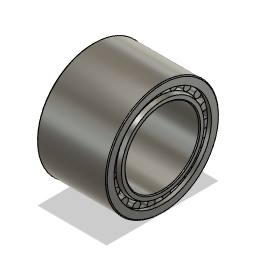
Bearing_GOST_7634-75_452000 (Autodesk Fusion 360 design; units mm, degrees)
Autodesk Fusion 360 part; units mm, degrees
note: some values were not read from the file. Chosen so that the rebuilt part matches the saved one: which bodies a step acts on.
sketch "Sketch1" plane through (0, 0, 0) normal (0, 0, 1) x (1, 0, 0)
  line L0 (-45.3984, 0) -> (45.3984, 0)
  line L1 (-80, 130) -> (80, 130)
  line L2 (80, 130) -> (80, 116.5)
  line L3 (80, 116.5) -> (-80, 116.5)
  line L4 (-80, 116.5) -> (-80, 130)
  line L5 (-80, 116.5) -> (-70.8611, 116.5)
  line L6 (-70.8611, 116.5) -> (-70.8611, 112)
  line L7 (-70.8611, 112) -> (-80, 112)
  line L8 (-80, 112) -> (-80, 116.5)
  line L9 (80, 116.5) -> (70.8611, 116.5)
  line L10 (70.8611, 116.5) -> (70.8611, 112)
  line L11 (70.8611, 112) -> (80, 112)
  line L12 (80, 112) -> (80, 116.5)
  line L13 (-80, 85) -> (80, 85)
  line L14 (-80, 85) -> (-80, 95.1737)
  line L15 (-80, 95.1737) -> (-70.8611, 98.5)
  line L16 (-70.8611, 98.5) -> (70.8611, 98.5)
  line L17 (80, 85) -> (80, 95.1737)
  line L18 (80, 95.1737) -> (70.8611, 98.5)
  line L19 (-70.8611, 98.5) -> (-70.8611, 112)
  line L20 (70.8611, 98.5) -> (70.8611, 112)
  line L21 (0, 98.5) -> (0, 85) construction
  line L22 (-70.8611, 107.5) -> (70.8611, 107.5)
  line L23 (-53.5833, 116.5) -> (-53.5833, 98.5)
  line L24 (0, 116.5) -> (0, 98.5)
  line L25 (-53.0833, 116.5) -> (-53.0833, 98.5)
  line L26 (-35.8056, 116.5) -> (-35.8056, 98.5)
  line L27 (-35.3056, 116.5) -> (-35.3056, 98.5)
  line L28 (-18.0278, 116.5) -> (-18.0278, 98.5)
  line L29 (-17.5278, 116.5) -> (-17.5278, 98.5)
  line L30 (-0.25, 116.5) -> (-0.25, 98.5)
  line L31 (0, 116.5) -> (0, 98.5)
  line L32 (17.5278, 116.5) -> (17.5278, 98.5)
  line L33 (18.0278, 116.5) -> (18.0278, 98.5)
  line L34 (35.3056, 116.5) -> (35.3056, 98.5)
  line L35 (35.8056, 116.5) -> (35.8056, 98.5)
  line L36 (53.0833, 116.5) -> (53.0833, 98.5)
  line L37 (53.5833, 116.5) -> (53.5833, 98.5)
  line L38 (0.25, 116.5) -> (0.25, 98.5)
  point P0 (0, 130)
  point P1 (0, 107.5)
  point P2 (0, 107.5)
  dimension "d1" = 170
  dimension "d2" = 20
  dimension "d3" = 20
  dimension "d4" = 260
  dimension "d5" = 160
  dimension "d7" = 18
  dimension "d8" = 9.1389
  dimension "d9" = 9
  dimension "d10" = 17.2778
  dimension "d23" = 0.5
  dimension "d24" = 17.2778
  dimension "d25" = 0.5
  dimension "d26" = 17.2778
  dimension "d27" = 0.5
  dimension "d28" = 17.2778
  dimension "d30" = 0.5
  dimension "d31" = 17.2778
  dimension "d32" = 0.5
  dimension "d33" = 17.2778
  dimension "d34" = 0.5
  dimension "d35" = 0.5
  dimension "d36" = 17.2778
  constraint horizontal L0
  constraint midpoint L0 origin
  constraint horizontal L1
  constraint vertical L2
  constraint horizontal L3
  constraint vertical L4
  constraint horizontal L5
  constraint vertical L6
  constraint horizontal L7
  constraint vertical L8
  constraint horizontal L9
  constraint vertical L10
  constraint horizontal L11
  constraint vertical L12
  constraint midpoint L1 P0
  constraint vertical origin P0
  constraint equal L7 L11
  constraint horizontal L13
  constraint vertical L1.end L13.end
  constraint vertical L1.start L13.start
  constraint perpendicular L13 L14
  constraint perpendicular L14 L16
  constraint perpendicular L13 L17
  constraint vertical L6.end L15.end
  constraint vertical L10.end L16.end
  constraint perpendicular L16 L19
  constraint perpendicular L11 L20
  constraint horizontal L6.end L10.end
  constraint midpoint L16 L21.start
  constraint midpoint L13 L21.end
  constraint equal L4 L21
  constraint coincident L22 P2
  constraint coincident L20 L22.end
  constraint coincident L19 L22.start
  constraint coincident L3 L23.start
  constraint coincident L16 L23.end
  constraint perpendicular L16 L23
  constraint midpoint L22 P2
  constraint midpoint L3 L24.start
  constraint midpoint L24 P2
  constraint coincident P2 P1
  constraint coincident L3 L25.start
  constraint coincident L16 L25.end
  constraint perpendicular L16 L25
  constraint coincident L3 L26.start
  constraint coincident L16 L26.end
  constraint perpendicular L16 L26
  constraint coincident L3 L27.start
  constraint coincident L16 L27.end
  constraint perpendicular L3 L27
  constraint coincident L3 L28.start
  constraint coincident L16 L28.end
  constraint perpendicular L16 L28
  constraint coincident L3 L29.start
  constraint coincident L16 L29.end
  constraint perpendicular L3 L29
  constraint coincident L3 L30.start
  constraint coincident L16 L30.end
  constraint perpendicular L16 L30
  constraint coincident L3 L24.start
  constraint coincident L16 L21.start
  constraint perpendicular L16 L31
  constraint coincident L24.start L31.start
  constraint coincident L3 L32.start
  constraint coincident L16 L32.end
  constraint perpendicular L16 L32
  constraint coincident L3 L33.start
  constraint coincident L16 L33.end
  constraint perpendicular L16 L33
  constraint coincident L3 L34.start
  constraint coincident L16 L34.end
  constraint perpendicular L16 L34
  constraint coincident L3 L35.start
  constraint coincident L16 L35.end
  constraint perpendicular L16 L35
  constraint coincident L3 L36.start
  constraint coincident L16 L36.end
  constraint perpendicular L16 L36
  constraint coincident L3 L37.start
  constraint coincident L16 L37.end
  constraint perpendicular L16 L37
  constraint coincident L3 L38.start
  constraint coincident L16 L38.end
  constraint perpendicular L16 L38
  measures "d2" angle of L16 L18
  measures "d3" angle of L15 L16
  measures "d5" distance of L1.start L1.end
  measures "d7" distance of L3 L16
  measures "d8" distance of L6.end L7.end
  measures "d10" distance of L19 L23
  measures "d23" distance of L23 L25
  measures "d24" distance of L25 L26
  measures "d25" distance of L26 L27
  measures "d26" distance of L27 L28
  measures "d27" distance of L28 L29
  measures "d28" distance of L29 L30
  measures "d30" distance of L32 L33
  measures "d31" distance of L33 L34
  measures "d32" distance of L34 L35
  measures "d33" distance of L35 L36
  measures "d34" distance of L36 L37
  measures "d35" distance of L30 L38
  measures "d36" distance of L32 L38
revolve "Revolve1" add sketch "Sketch1" angle 360 about axis through (-45.3984, 0, 0) along (1, 0, 0) contours L1 L2 L3 L4 L5 L9 | L3 L5 L6 L7 L8 | L3 L9 L10 L11 L12 | L13 L14 L15 L16 L17 L18 makes body 1 at (-23.6204, 98.3776, -4.9098) makes body 2 at (-26.6667, 129.8384, -6.48)
revolve "Revolve2" add sketch "Sketch1" angle 360 about axis through (-70.8611, 107.5, 0) along (1, 0, 0) separate body contours L16 L19 L22 L23 | L16 L20 L22 L37 | L16 L22 L25 L26 | L16 L22 L35 L36 | L16 L22 L27 L28 | L16 L22 L33 L34 | L16 L22 L29 L30 | L16 L22 L32 L38 makes body 3 at (-65.1019, 98.5112, 0.4486) makes body 4 at (65.1019, 98.5112, 0.4486) makes body 5 at (23.787, 98.5112, 0.4486) makes body 6 at (-11.7685, 98.5447, 0.8961) makes body 7 at (-29.5463, 98.5112, 0.4486) makes body 8 at (47.3241, 98.5447, 0.8961) makes body 9 at (6.0093, 98.5112, 0.4486) makes body 10 at (-47.3241, 98.5112, 0.4486)
pattern_circular "C-Pattern1" count 19 over 360 about axis through (-45.3984, 0, 0) along (1, 0, 0) of "Revolve2" makes body 11 at (-65.1019, 53.5049, 82.7156) makes body 12 at (65.1019, 53.5049, 82.7156) makes body 13 at (-65.1019, 23.7482, 95.6069) makes body 14 at (65.1019, 23.7482, 95.6069) makes body 15 at (-65.1019, -8.5821, 98.1377) makes body 16 at (65.1019, -8.5821, 98.1377) makes body 17 at (-65.1019, -39.9823, 90.0337) makes body 18 at (65.1019, -39.9823, 90.0337) makes body 19 at (-65.1019, -67.0499, 72.1732) makes body 20 at (65.1019, -97.2415, 15.7719) makes body 21 at (-65.1019, -97.0938, -16.6569) makes body 22 at (65.1019, -97.0938, -16.6569) makes body 23 at (65.1019, -66.3898, -72.7809) makes body 24 at (-65.1019, 54.2561, -82.2249) makes body 25 at (65.1019, 54.2561, -82.2249) makes body 26 at (-47.3241, 93.0279, 32.4108) makes body 27 at (-11.7685, 77.2152, 61.2346) makes body 28 at (-11.7685, -87.094, 46.114) makes body 29 at (-47.3241, -86.4245, -47.2807) makes body 30 at (-11.7685, -38.7643, -90.6046) makes body 31 at (6.0093, -7.6879, -98.2118) makes body 32 at (-6.0093, 25.06, -95.3093) makes body 33 at (-11.7685, 78.316, -59.8203) makes body 34 at (6.0093, 93.3192, -31.5622) makes body 35 at (41.5648, 93.0279, 32.4108) makes body 36 at (65.1019, 77.4636, 60.8608) makes body 37 at (47.3241, -67.4018, 71.8948) makes body 38 at (65.1019, -86.8515, 46.4916) makes body 39 at (11.7685, -97.3482, 15.336) makes body 40 at (47.3241, -86.241, -47.6902) makes body 41 at (11.7685, -66.0832, -73.1086) makes body 42 at (41.5648, -39.1607, -90.3941) makes body 43 at (-47.3241, -7.6879, -98.2118) makes body 44 at (47.3241, 25.06, -95.3093) makes body 45 at (47.3241, 78.316, -59.8203) makes body 46 at (41.5648, 93.3192, -31.5622) makes body 47 at (23.787, 93.0279, 32.4108) makes body 48 at (-11.7685, 92.9143, 32.845) makes body 49 at (-29.5463, 93.0279, 32.4108) makes body 50 at (6.0093, 93.0279, 32.4108) makes body 51 at (-65.1019, 93.0279, 32.4108) makes body 52 at (65.1019, 93.0279, 32.4108) makes body 53 at (23.787, 77.4636, 60.8608) makes body 54 at (-29.5463, 77.4636, 60.8608) makes body 55 at (41.5648, 77.4636, 60.8608) makes body 56 at (11.7685, 77.2152, 61.2346) makes body 57 at (-65.1019, 77.4636, 60.8608) makes body 58 at (-47.3241, 77.4636, 60.8608) makes body 59 at (23.787, 53.5049, 82.7156) makes body 60 at (-11.7685, 53.1487, 82.9885) makes body 61 at (-23.787, 53.1487, 82.9885) makes body 62 at (47.3241, 53.1487, 82.9885) makes body 63 at (11.7685, 53.1487, 82.9885) makes body 64 at (-47.3241, 53.5049, 82.7156) makes body 65 at (23.787, 23.7482, 95.6069) makes body 66 at (-11.7685, 23.3226, 95.7493) makes body 67 at (-29.5463, 23.7482, 95.6069) makes body 68 at (47.3241, 23.3226, 95.7493) makes body 69 at (6.0093, 23.7482, 95.6069) makes body 70 at (-41.5648, 23.3226, 95.7493) makes body 71 at (23.787, -8.5821, 98.1377) makes body 72 at (-11.7685, -9.0308, 98.1341) makes body 73 at (-29.5463, -8.5821, 98.1377) makes body 74 at (47.3241, -9.0308, 98.1341) makes body 75 at (6.0093, -8.5821, 98.1377) makes body 76 at (-47.3241, -8.5821, 98.1377) makes body 77 at (23.787, -39.9823, 90.0337) makes body 78 at (-11.7685, -40.4056, 89.8847) makes body 79 at (-29.5463, -39.9823, 90.0337) makes body 80 at (47.3241, -40.4056, 89.8847) makes body 81 at (11.7685, -40.4056, 89.8847) makes body 82 at (-47.3241, -39.9823, 90.0337) makes body 83 at (29.5463, -67.4018, 71.8948) makes body 84 at (-11.7685, -67.4018, 71.8948) makes body 85 at (-29.5463, -67.0499, 72.1732) makes body 86 at (11.7685, -67.4018, 71.8948) makes body 87 at (-47.3241, -67.0499, 72.1732) makes body 88 at (65.1019, -67.0499, 72.1732) makes body 89 at (23.787, -86.8515, 46.4916) makes body 90 at (-29.5463, -86.8515, 46.4916) makes body 91 at (47.3241, -87.094, 46.114) makes body 92 at (11.7685, -87.094, 46.114) makes body 93 at (-65.1019, -86.8515, 46.4916) makes body 94 at (-41.5648, -87.094, 46.114) makes body 95 at (23.787, -97.2415, 15.7719) makes body 96 at (-11.7685, -97.3482, 15.336) makes body 97 at (-29.5463, -97.2415, 15.7719) makes body 98 at (47.3241, -97.3482, 15.336) makes body 99 at (-65.1019, -97.2415, 15.7719) makes body 100 at (-47.3241, -97.2415, 15.7719) makes body 101 at (23.787, -97.0938, -16.6569) makes body 102 at (-11.7685, -97.0532, -17.1038) makes body 103 at (-29.5463, -97.0938, -16.6569) makes body 104 at (47.3241, -97.0532, -17.1038) makes body 105 at (6.0093, -97.0938, -16.6569) makes body 106 at (-47.3241, -97.0938, -16.6569) makes body 107 at (23.787, -86.4245, -47.2807) makes body 108 at (-6.0093, -86.241, -47.6902) makes body 109 at (-23.787, -86.241, -47.6902) makes body 110 at (11.7685, -86.241, -47.6902) makes body 111 at (-65.1019, -86.241, -47.6902) makes body 112 at (65.1019, -86.4245, -47.2807) makes body 113 at (23.787, -66.3898, -72.7809) makes body 114 at (-11.7685, -66.0832, -73.1086) makes body 115 at (-29.5463, -66.3898, -72.7809) makes body 116 at (47.3241, -66.0832, -73.1086) makes body 117 at (-65.1019, -66.3898, -72.7809) makes body 118 at (-47.3241, -66.3898, -72.7809) makes body 119 at (23.787, -39.1607, -90.3941) makes body 120 at (-29.5463, -39.1607, -90.3941) makes body 121 at (6.0093, -39.1607, -90.3941) makes body 122 at (-65.1019, -39.1607, -90.3941) makes body 123 at (-41.5648, -38.7643, -90.6046) makes body 124 at (65.1019, -39.1607, -90.3941) makes body 125 at (23.787, -7.6879, -98.2118) makes body 126 at (-11.7685, -7.2447, -98.2821) makes body 127 at (-29.5463, -7.6879, -98.2118) makes body 128 at (47.3241, -7.2447, -98.2821) makes body 129 at (-65.1019, -7.6879, -98.2118) makes body 130 at (65.1019, -7.6879, -98.2118) makes body 131 at (23.787, 24.618, -95.3866) makes body 132 at (-29.5463, 24.618, -95.3866) makes body 133 at (11.7685, 25.06, -95.3093) makes body 134 at (-65.1019, 25.06, -95.3093) makes body 135 at (-47.3241, 24.618, -95.3866) makes body 136 at (65.1019, 24.618, -95.3866) makes body 137 at (23.787, 54.2561, -82.2249) makes body 138 at (-11.7685, 54.649, -82.0082) makes body 139 at (-29.5463, 54.2561, -82.2249) makes body 140 at (47.3241, 54.649, -82.0082) makes body 141 at (11.7685, 54.649, -82.0082) makes body 142 at (-47.3241, 54.2561, -82.2249) makes body 143 at (23.787, 78.0147, -60.1528) makes body 144 at (-29.5463, 78.0147, -60.1528) makes body 145 at (11.7685, 78.316, -59.8203) makes body 146 at (-65.1019, 78.0147, -60.1528) makes body 147 at (-47.3241, 87.1563, -74.7227) makes body 148 at (65.1019, 78.0147, -60.1528) makes body 149 at (23.787, 93.3192, -31.5622) makes body 150 at (-11.7685, 93.4963, -31.1499) makes body 151 at (-29.5463, 93.3192, -31.5622) makes body 152 at (-65.1019, 93.3192, -31.5622) makes body 153 at (-41.5648, 93.4963, -31.1499) makes body 154 at (65.1019, 93.3192, -31.5622)
fillet "Fillet1" radius 2 4 edges at (-80, -30.7373, 79.2478) (80, -30.7373, 79.2478) (-80, -47.01, 121.2026) (80, -47.01, 121.2026) on bodies 1 2
